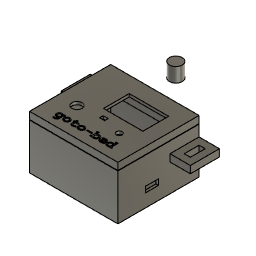
goto-bed (Autodesk Fusion 360 design; units mm, degrees)
Autodesk Fusion 360 part; units mm, degrees
sketch "top" plane through (0, 0, 0) normal (0, 0, 1) x (1, 0, 0)
  line L0 (28.55, -26.05) -> (-28.55, -26.05)
  line L1 (-28.55, -26.05) -> (-28.55, 26.05)
  line L2 (-28.55, 26.05) -> (28.55, 26.05)
  line L3 (28.55, 26.05) -> (28.55, -26.05)
  line L4 (28.55, -26.05) -> (-28.55, 26.05) construction
  line L5 (-28.55, -26.05) -> (28.55, 26.05) construction
  line L6 (30.85, -28.35) -> (-30.85, -28.35)
  line L7 (-30.85, -28.35) -> (-30.85, 28.35)
  line L8 (-30.85, 28.35) -> (30.85, 28.35)
  line L9 (30.85, 28.35) -> (30.85, -28.35)
  line L10 (-6.75, 17.2) -> (20.75, 17.2)
  line L11 (20.75, 17.2) -> (20.75, -0.8)
  line L12 (20.75, -0.8) -> (-6.75, -0.8)
  line L13 (-6.75, -0.8) -> (-6.75, 17.2)
  line L14 (-2.5, -5.3) -> (1, -5.3)
  line L15 (1, -5.3) -> (1, -7.7)
  line L16 (1, -7.7) -> (-2.5, -7.7)
  line L17 (-2.5, -7.7) -> (-2.5, -5.3)
  circle A0 centre (13.75, -10.3) radius 2
  circle A1 centre (-17.75, -8.3) radius 3.5
  line L18 (26.25, -23.75) -> (-26.25, -23.75)
  line L19 (-26.25, -23.75) -> (-26.25, 23.75)
  line L20 (-26.25, 23.75) -> (26.25, 23.75)
  line L21 (26.25, 23.75) -> (26.25, -23.75)
  line L22 (0, 28.35) -> (0, -28.35) construction
  line L23 (-20.6534, -23.35) -> (20.6534, -23.35) construction
  line L24 (20.6534, -23.35) -> (20.6534, -15.8454) construction
  line L25 (20.6534, -15.8454) -> (-20.6534, -15.8454) construction
  line L26 (-20.6534, -15.8454) -> (-20.6534, -23.35) construction
  dimension "d1" = 57.1
  dimension "d2" = 52.1
  dimension "d3" = -2.3
  dimension "d4" = 27.5
  dimension "d5" = 18
  dimension "d10" = 3.5
  dimension "d11" = 2.4
  dimension "d12" = 4.5
  dimension "d13" = 4.25
  dimension "d14" = 4
  dimension "d15" = 7
  dimension "d16" = 25.25
  dimension "d21" = 7.5
  dimension "d22" = 10.75
  dimension "d60" = 2.3
  dimension "d185" = 5.5
  dimension "d186" = 7.5
  dimension "d187" = 4
  text T0 "goto-bed" font "Courier New" height 5 bold align centre middle in box 41.3068 x 7.5046 at (-20.6534, -23.35) x (1, 0) y (0, 1) spacing 1 kerned
  constraint horizontal L0
  constraint perpendicular L0 L1
  constraint parallel L0 L2
  constraint parallel L1 L3
  constraint coincident L4 origin
  constraint coincident L5 origin
  constraint horizontal L10
  constraint vertical L11
  constraint horizontal L12
  constraint vertical L13
  constraint horizontal L14
  constraint vertical L15
  constraint horizontal L16
  constraint vertical L17
  constraint midpoint L8 L22.start
  constraint midpoint L6 L22.end
  constraint perpendicular L22 L25
  constraint coincident L22
  measures "d1" distance of L1.end L2.end
  measures "d2" distance of L0.end L1.end
  measures "d4" distance of L10.start L10.end
  measures "d5" distance of L10.start L12.end
  measures "d10" distance of L14.start L14.end
  measures "d11" distance of L14.start L16.end
  measures "d12" distance of L12 L14
  measures "d13" distance of L12.end L17
  measures "d14" diameter of A0
  measures "d15" diameter of A1
  measures "d16" distance of L0 L12
  measures "d21" distance of L12 A0
  measures "d22" distance of L15 A0
  measures "d185" distance of L11 L21
  measures "d186" distance of L13 A1
  measures "d187" distance of L12 A1
extrude "Extrude2" add sketch "top" against normal blind 2 contours L0 L1 L2 L3 | L6 L7 L8 L9 | L18 L19 L20 L21 makes body 1
extrude "Extrude3" add sketch "top" against normal blind 5 contours L6 L7 L8 L9 bodies 1
extrude "Extrude8" add sketch "top" against normal blind 13 contours L0 L1 L2 L3 bodies 1
sketch "bottom" plane through (0, 0, -5) normal (0, 0, -1) x (1, 0, 0)
  line L0 (26.35, -22.5) -> (-26.35, -22.5)
  line L1 (-26.35, -22.5) -> (-26.35, 22.5)
  line L2 (-26.35, 22.5) -> (26.35, 22.5)
  line L3 (28.65, 24.8) -> (-28.65, 24.8)
  circle A0 centre (0, 0) radius 5.25
  line L4 (28.55, -26.05) -> (-28.55, -26.05)
  line L5 (-28.55, -26.05) -> (-28.55, 26.05)
  line L6 (-28.55, 26.05) -> (28.55, 26.05)
  line L7 (28.55, 26.05) -> (28.55, -26.05)
  line L8 (-30.85, -28.35) -> (30.85, -28.35)
  line L9 (30.85, -28.35) -> (30.85, 28.35)
  line L10 (30.85, 28.35) -> (-30.85, 28.35)
  line L11 (-30.85, 28.35) -> (-30.85, -28.35)
  line L12 (0, 0) -> (5.25, 0) construction
  line L13 (5.25, 0) -> (7.75, 0) construction
  line L14 (0, -2) -> (7.75, -2)
  arc A1 (7.75, -2) -> (7.75, 2) centre (7.75, 0) ccw
  line L15 (7.75, 2) -> (0, 2)
  arc A2 (0, 2) -> (0, -2) centre (0, 0) ccw
  line L16 (0, 0) -> (7.75, 0) construction
  line L17 (45.1, -8.03) -> (30.85, -8.03)
  line L18 (30.85, -8.03) -> (30.85, -28.35)
  line L19 (30.85, -28.35) -> (45.1, -28.35)
  line L20 (45.1, -28.35) -> (45.1, -8.03)
  line L21 (45.1, -8.03) -> (30.85, -28.35) construction
  line L22 (30.85, -8.03) -> (45.1, -28.35) construction
  line L23 (40.1, -13.03) -> (35.85, -13.03)
  line L24 (35.85, -13.03) -> (35.85, -23.35)
  line L25 (35.85, -23.35) -> (40.1, -23.35)
  line L26 (40.1, -23.35) -> (40.1, -13.03)
  line L27 (0, -28.35) -> (0, 28.35) construction
  line L28 (-30.85, -28.35) -> (-45.1, -28.35)
  line L29 (-45.1, -28.35) -> (-45.1, -8.03)
  line L30 (-45.1, -8.03) -> (-30.85, -8.03)
  line L31 (-30.85, -8.03) -> (-30.85, -28.35)
  line L32 (-35.85, -13.03) -> (-35.85, -23.35)
  line L33 (-40.1, -23.35) -> (-40.1, -13.03)
  line L34 (-40.1, -13.03) -> (-35.85, -13.03)
  line L35 (-35.85, -23.35) -> (-40.1, -23.35)
  line L36 (-21.2881, 24.9708) -> (21.5542, 24.6038) construction
  line L37 (21.5542, 24.6038) -> (21.4211, 9.0755) construction
  line L38 (21.4211, 9.0755) -> (-21.4211, 9.4424) construction
  line L39 (-21.4211, 9.4424) -> (-21.2881, 24.9708) construction
  point P0 (37.975, -18.19)
  point P1 (30.85, -18.19)
  point P2 (30.85, -28.35)
  dimension "d67" = 10.5
  dimension "d131" = 2.5
  dimension "d132" = 2
  dimension "d192" = 14.25
  dimension "d193" = 20.32
  dimension "d194" = -5
  text T0 "Barrett Otte\n2021" font "Courier New" height 3 bold align centre middle in box 42.8439 x 15.529 at (-21.2881, 24.9708) x (0.999963, -0.008565) y (-0.008565, -0.999963) spacing 1 kerned mirrored across
  constraint coincident A0.centre L12.start
  constraint horizontal L12
  constraint coincident A0 L12.end
  constraint parallel L12 L13
  constraint tangent L14 A1
  constraint tangent A1 L15
  constraint parallel L14 L15
  constraint tangent L15 A2
  constraint tangent L14 A2
  constraint coincident L13.end A1.centre
  constraint parallel L13 L16
  constraint horizontal L17
  constraint perpendicular L17 L18
  constraint parallel L17 L19
  constraint parallel L18 L20
  constraint coincident L21 P0
  constraint coincident L22 P0
  constraint coincident L18 P1
  constraint horizontal P0 P1
  constraint midpoint L8 L27.start
  constraint midpoint L10 L27.end
  constraint symmetric L17.start L27 L29.end
  constraint symmetric L17.end L27 L30.end
  constraint symmetric P2 L27 L8.start
  constraint symmetric L19.end L27 L28.end
  constraint symmetric L23.start L27 L33.end
  constraint symmetric L23.end L27 L32.start
  constraint symmetric L24.end L27 L32.end
  constraint symmetric L25.end L27 L33.start
  constraint coincident L27
  constraint coincident L19 P2
  constraint coincident L18 P2
  measures "d67" diameter of A0
  measures "d131" distance of L12.end L13.end
  measures "d132" radius of A1
  measures "d192" distance of P2 L19.end
  measures "d193" distance of L17.end P2
extrude "Extrude9" add sketch "bottom" along normal blind 32 from surface at 0.25 separate body contours L8 L9 L10 L11 L18 L31 makes body 2
extrude "Extrude10" add sketch "bottom" along normal blind 2.5 from surface at 29.75 contours L3 L4 L5 L7 | L3 L5 L6 L7 bodies 2
sketch "bottom_backplate" plane through (0, 0, -34.75) normal (0, 0, 1) x (-1, 0, 0)
  line L0 (-4.8541, -2) -> (-7.75, -2)
  arc A0 (-7.75, 2) -> (-7.75, -2) centre (-7.75, 0) ccw
  line L1 (-7.75, 2) -> (-4.8541, 2)
  line L2 (-28.55, 26.05) -> (-28.55, -26.05)
  line L3 (-28.55, -26.05) -> (28.55, -26.05)
  line L4 (28.55, 26.05) -> (-28.55, 26.05)
  line L5 (28.55, -26.05) -> (-28.55, -26.05)
  line L6 (-28.55, -26.05) -> (-28.55, 26.05)
  line L7 (-28.55, 26.05) -> (28.55, 26.05)
  line L8 (28.55, 26.05) -> (28.55, -26.05)
  line L9 (-4.8541, -2) -> (-4.8541, 2)
  line L10 (-4.8541, -2) -> (-7.75, -2)
  line L11 (-4.8541, 2) -> (-7.75, 2)
  arc A1 (-7.75, 2) -> (-7.75, -2) centre (-7.75, 0) ccw
  line L12 (28.55, -26.05) -> (28.55, 26.05)
  dimension "d137" = 2
  constraint horizontal L5
  constraint vertical L6
  constraint horizontal L7
  constraint vertical L8
  constraint coincident L2.start L4.end
  constraint coincident L3.end L5.start
  constraint coincident L0.start L9.start
  constraint coincident L1.end L9.end
  constraint coincident L0.end A0.end
  constraint coincident A0.start L1.start
  measures "d137" radius of A1
extrude "Extrude11" add sketch "bottom_backplate" along normal blind 3 bodies 2
sketch "right" plane through (30.85, 0, 0) normal (1, 0, 0) x (0, 1, 0)
  line L0 (28.35, -5.25) -> (-28.35, -5.25)
  line L1 (-28.35, -5.25) -> (-28.35, -37.25)
  line L2 (-28.35, -37.25) -> (28.35, -37.25)
  line L3 (28.35, -37.25) -> (28.35, -5.25)
  line L4 (0, -24.15) -> (-9, -24.15)
  line L5 (-9, -24.15) -> (-9, -28.15)
  line L6 (-9, -28.15) -> (0, -28.15)
  line L7 (0, -28.15) -> (0, -24.15)
  line L8 (0, -24.15) -> (-9, -28.15) construction
  line L9 (-9, -24.15) -> (0, -28.15) construction
  line L10 (26.05, -5) -> (-26.05, -5)
  line L11 (-26.05, -5) -> (-26.05, -13)
  line L12 (-26.05, -13) -> (26.05, -13)
  line L13 (26.05, -13) -> (26.05, -5)
  line L14 (28.35, 0) -> (-28.35, 0)
  line L15 (-28.35, 0) -> (-28.35, -5)
  line L16 (-28.35, -5) -> (28.35, -5)
  line L17 (28.35, -5) -> (28.35, 0)
  line L18 (17.2, 0) -> (17.2, -2)
  line L19 (17.2, -2) -> (-0.8, -2)
  line L20 (-0.8, -2) -> (-0.8, 0)
  line L21 (-2, -34.75) -> (2, -34.75)
  line L22 (2, -34.75) -> (2, -31.75)
  line L23 (2, -31.75) -> (-2, -31.75)
  line L24 (-2, -31.75) -> (-2, -34.75)
  line L25 (-0.8, 0) -> (17.2, 0)
  line L26 (0, 0) -> (0, -37.25) construction
  point P0 (-4.5, -26.15)
  point P1 (0, -26.15)
  dimension "d140" = 9
  dimension "d141" = 4
  dimension "d145" = 24.15
  dimension "d146" = 0.8
  constraint horizontal L4
  constraint perpendicular L4 L5
  constraint parallel L4 L6
  constraint parallel L5 L7
  constraint coincident L8 P0
  constraint coincident L9 P0
  constraint coincident L26.start origin
  constraint midpoint L2 L26.end
  constraint midpoint L7 P1
  constraint coincident L26 P1
  measures "d140" distance of L5.end L6.end
  measures "d141" distance of L4.end L5.end
  measures "d145" distance of L4 L14
extrude "Extrude12" cut sketch "right" against normal blind 3 contours L4 L5 L6 L7 bodies 2
extrude "Extrude16" cut sketch "top" against normal blind 1.5 text T0 bodies 1
extrude "Extrude17" add sketch "bottom" along normal blind 5 from surface at 8 contours L11 L28 L29 L30 L31 | L9 L17 L18 L19 L20 bodies 2
extrude "Extrude18" cut sketch "bottom" against normal blind 1.5 from surface at 32.25 text T0 bodies 2
move_face "OffsetFaces1" offset -0.5 4 faces at (-9.5167, -26.05, -14.0833) (28.55, 0, -11.55) (-28.55, 8.6833, -14.0833) (9.5167, 26.05, -14.0833) on bodies 2
sketch "pot-dial" plane through (0, 0, 0) normal (0, 0, 1) x (1, 0, 0)
  circle A0 centre (0, 0) radius 4.5
  line L0 (0, -4.5) -> (0, 4.5) construction
  point P0 (0, -4.5)
  point P1 (3, -6.5)
  point P2 (0, 4.5)
  dimension "d202" = 9
  constraint coincident A0.centre origin
  constraint vertical L0
  constraint coincident A0 P0
  constraint coincident L0 P0
  constraint coincident A0 P2
  constraint coincident L0 P2
  constraint coincident P0 L0.start
  constraint coincident P2 L0.end
  measures "d202" diameter of A0
extrude "Extrude19" add sketch "pot-dial" along normal blind 8 separate body makes body 3
extrude "Extrude20" add 1 faces at (0.9352, 1.1727, 8) along direction (0, 0, 1) blind 2 on bodies 3 bodies 3
shell "Shell1" thickness 1.5 removed faces 1 at (0.9352, 1.1727, 0) on bodies 3
move_body "Move1" bodies 3 to x (1, 0, 0) y (0, 1, 0) z (0, 0, 1) at (0, 43, 0)
named bodies: "top", "bottom", "pot-dial"
